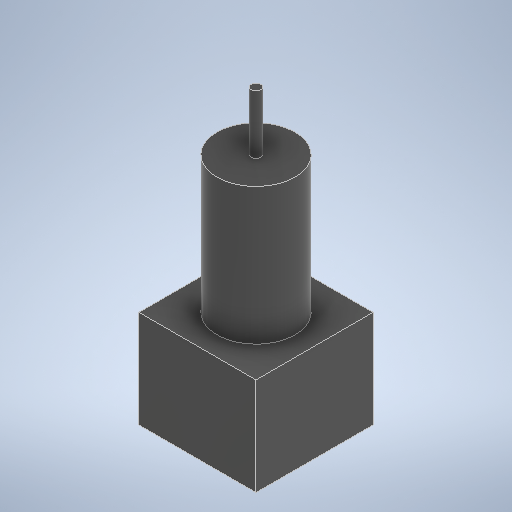
# Autodesk Inventor part: Herramienta
Saved by Autodesk Inventor 2025 (Build 290162000, 162)
## iProperties
Created: 2023-05-06
Part Number: Herramienta
Material: Hierro, fundido
Document SubType Name: Modeling
Designer: Miguel Ángel
Density: 7.15 g/cm^3
Appearance: Gris oscuro
Author: Miguel Ángel
Autodesk Inventor part; units mm, degrees
ref_plane "YZ Plane" through (0, 0, 0) normal (1, 0, 0) x (0, 1, 0)
ref_plane "XZ Plane" through (0, 0, 0) normal (0, 1, 0) x (-1, 0, 0)
ref_plane "XY Plane" through (0, 0, 0) normal (0, 0, 1) x (1, 0, 0)
sketch "Boceto1" plane through (0, 0, 0) normal (0, 1, 0) x (-1, 0, 0)
  line L0 (-3, 3) -> (3, 3)
  line L1 (3, 3) -> (3, -3)
  line L2 (3, -3) -> (-3, -3)
  line L3 (-3, -3) -> (-3, 3)
  line L4 (-3, 3) -> (3, -3) construction
  line L5 (3, 3) -> (-3, -3) construction
  point P0 (0, 0)
  dimension "d0" = 6
  dimension "d1" = 6
  constraints: 12 end point, 2 midpoint, 2 parallel, 1 horizontal, 1 perpendicular
  measures "d0" distance of L1.end L2.end
  measures "d1" distance of L0.end L1.end
extrude "Extrusión1" add sketch "Boceto1" along normal blind 5
sketch "Boceto2" plane through (0, 5, 0) normal (0, 1, 0) x (1, 0, 0)
  circle A0 centre (0, 0) radius 2
  dimension "d4" = 4
  constraints: 1 centre point, 1 coincident
  measures "d4" diameter of A0
extrude "Extrusión2" add sketch "Boceto2" along normal blind 7
sketch "Boceto3" plane through (0, 12, 0) normal (0, 1, 0) x (1, 0, 0)
  circle A0 centre (0, 0) radius 0.25
  dimension "d7" = 0.5
  constraints: 1 centre point, 1 coincident
  measures "d7" diameter of A0
extrude "Extrusión3" add sketch "Boceto3" along normal blind 3
